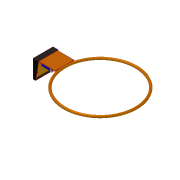
# Autodesk Inventor part: GE-12013
Saved by Autodesk Inventor 2012 (Build 160160000, 160)
## iProperties
Created: 2011-05-25
Part Number: GE-12013
Document SubType Name: Modeling
Designer: dfoster
Density: 1 g/cm^3
Description: Basketball Hoop
Mass: 471.421 g
Surface Area: 1803.58 cm^2
Volume: 471.421 cm^3
Material: Default
Title: Basketball Hoop
Author: dfoster
Autodesk Inventor part; units mm, degrees
ref_plane "YZ Plane" through (0, 0, 0) normal (1, 0, 0) x (0, 1, 0)
ref_plane "XZ Plane" through (0, 0, 0) normal (0, 1, 0) x (-1, 0, 0)
ref_plane "XY Plane" through (0, 0, 0) normal (0, 0, 1) x (1, 0, 0)
sketch "Sketch1" plane through (0, 0, 0) normal (0, 0, 1) x (1, 0, 0)
  circle A0 centre (0, 0) radius 7.9375
  line L0 (236.5375, 47.7842) -> (236.5375, -114.9552)
  dimension "d0" = 228.6
  dimension "d1" = 15.875
  constraints: 2 end point, 1 centre point, 1 coincident, 1 vertical
  measures "d0" distance edge to line of A0 L0
  measures "d1" diameter of A0
revolve "Revolution1" add sketch "Sketch1" angle 360 about axis through (236.5375, 47.7842, 0) along (0, -1, 0)
sketch "Sketch2" plane through (0, 0, 0) normal (0, 0, 1) x (1, 0, 0)
  line L0 (0, 4.7625) -> (-134.9375, 4.7625)
  line L1 (-138.1125, 1.5875) -> (-138.1125, -106.3625)
  line L2 (-138.1125, -106.3625) -> (-141.2875, -106.3625)
  line L3 (-141.2875, -106.3625) -> (-141.2875, 1.5875)
  line L4 (-134.9375, 7.9375) -> (0, 7.9375)
  line L5 (0, 7.9375) -> (0, 4.7625)
  arc A0 (-134.9375, 4.7625) -> (-138.1125, 1.5875) centre (-134.9375, 1.5875) ccw
  arc A1 (-134.9375, 7.9375) -> (-141.2875, 1.5875) centre (-134.9375, 1.5875) ccw
  point P0 (0, 0)
  point P1 (-138.1125, 4.7625)
  dimension "d5" = 0
  dimension "d6" = 7.9375
  dimension "d7" = 3.175
  dimension "d8" = 3.175
  dimension "d9" = 6.35
  dimension "d27" = 114.3
  dimension "d28" = 141.2875
  constraints: 12 end point, 4 parallel, 4 point on circle, 4 tangent, 2 centre point, 2 perpendicular, 2 point on line, 1 horizontal
  measures "d5" distance from line of point (0, 0) L5
  measures "d6" distance from line of point (0, 0) L4
  measures "d7" distance between parallel lines of L0 L4
  measures "d8" radius of A0
  measures "d9" radius of A1
  measures "d27" distance between parallel lines of L2 L4
  measures "d28" distance between parallel lines of L5 L3
extrude "Extrusion1" add sketch "Sketch2" along normal mid plane 125.4125
sketch "Sketch3" plane through (-141.2875, -106.3625, 62.7062) normal (-1, 0, 0) x (0, 0, 1)
  line L0 (0, 0) -> (0, 107.95) projected
  line L1 (0, 107.95) -> (-125.4125, 107.95) projected
  line L2 (-125.4125, 107.95) -> (-125.4125, 0) projected
  line L3 (0, 0) -> (-125.4125, 0) projected
  line L4 (0, 114.3) -> (-125.4125, 114.3) projected
  line L5 (-125.4125, 107.95) -> (-125.4125, 114.3) projected
  line L6 (0, 114.3) -> (0, 107.95) projected
  arc A0 (-103.9113, 100.9746) -> (-110.4012, 84.7629) centre (-107.1562, 92.8687) ccw
  arc A1 (-102.47, 81.5879) -> (-95.9802, 97.7996) centre (-99.2251, 89.6937) ccw
  arc A2 (-29.4323, 97.7996) -> (-22.9425, 81.5879) centre (-26.1874, 89.6937) ccw
  arc A3 (-15.0113, 84.7629) -> (-21.5012, 100.9746) centre (-18.2562, 92.8687) ccw
  arc A4 (-110.4012, 31.1246) -> (-103.9113, 14.9129) centre (-107.1562, 23.0187) ccw
  arc A5 (-95.9802, 18.0879) -> (-102.47, 34.2996) centre (-99.2251, 26.1937) ccw
  arc A6 (-22.9425, 34.2996) -> (-29.4323, 18.0879) centre (-26.1874, 26.1937) ccw
  arc A7 (-21.5012, 14.9129) -> (-15.0113, 31.1246) centre (-18.2562, 23.0187) ccw
  line L7 (-110.4012, 84.7629) -> (-102.47, 81.5879)
  line L8 (-103.9113, 100.9746) -> (-95.9802, 97.7996)
  line L9 (-21.5012, 100.9746) -> (-29.4323, 97.7996)
  line L10 (-15.0113, 84.7629) -> (-22.9425, 81.5879)
  line L11 (-22.9425, 34.2996) -> (-15.0113, 31.1246)
  line L12 (-21.5012, 14.9129) -> (-29.4323, 18.0879)
  line L13 (-103.9113, 14.9129) -> (-95.9802, 18.0879)
  line L14 (-102.47, 34.2996) -> (-110.4012, 31.1246)
  line L15 (-107.1562, 23.0187) -> (-107.1562, 92.8687)
  line L16 (-99.2251, 26.1937) -> (-99.2251, 89.6937)
  line L17 (-26.1874, 26.1937) -> (-26.1874, 89.6937)
  line L18 (-18.2562, 23.0187) -> (-18.2562, 92.8687)
  line L19 (-99.2251, 89.6937) -> (-26.1874, 89.6937)
  line L20 (-107.1562, 92.8687) -> (-18.2562, 92.8687)
  line L21 (-99.2251, 26.1937) -> (-26.1874, 26.1937)
  line L22 (-107.1562, 23.0187) -> (-18.2562, 23.0187)
  dimension "d29" = 106.3625
  dimension "d30" = 55.5752
  dimension "d31" = 87.3125
  dimension "d32" = 46.0375
  dimension "d33" = 17.4625
  dimension "d34" = 9.525
  dimension "d35" = 12.7
  dimension "d36" = 9.525
  dimension "d37" = 33.3375
  dimension "d38" = 79.375
  dimension "d39" = 34.9186
  constraints: 32 end point, 16 point on circle, 14 tangent, 8 centre point, 7 equal radius, 4 horizontal, 4 vertical, 2 parallel, 1 coincident, 1 equal length
  measures "d33" distance between parallel lines of L7 L8
  measures "d34" distance edge to line of A0 L2
  measures "d35" distance edge to line of A3 L4
  measures "d36" distance edge to line of A3 L0
  measures "d38" distance edge to line of A6 L4
hole "Hole1" at (-138.1125, -15.0812, 40.4812) direction (-1, 0, 0) diameter 6.731 end through all
pattern_linear "Rectangular Pattern1" count 2 spacing 80.9625 along (0, 0, -1) count 2 spacing 66.675 along (0, -1, 0) of "Hole1"
hole "Hole2" at (-141.2875, -49.2125, 0.7937) direction (1, 0, 0) diameter 12.7 depth 25.4 tip angle 118
sketch "Sketch4" plane through (-141.2875, -106.3625, 62.7062) normal (-1, 0, 0) x (0, 0, 1)
  line L0 (0, 0) -> (0, 107.95) projected
  line L1 (-125.4125, 107.95) -> (-125.4125, 0) projected
  line L2 (0, 0) -> (-125.4125, 0) projected
  line L3 (-128.5875, -3.175) -> (3.175, -3.175)
  line L4 (3.175, -3.175) -> (3.175, 117.475)
  line L5 (3.175, 117.475) -> (-128.5875, 117.475)
  line L6 (-128.5875, 117.475) -> (-128.5875, -3.175)
  line L7 (0, 114.3) -> (-125.4125, 114.3) projected
  line L8 (-127, 115.8875) -> (1.5875, 115.8875)
  line L9 (1.5875, 115.8875) -> (1.5875, -1.5875)
  line L10 (1.5875, -1.5875) -> (-127, -1.5875)
  line L11 (-127, -1.5875) -> (-127, 115.8875)
  point P0 (-62.7062, 106.3625)
  dimension "d49" = 3.175
  dimension "d50" = 3.175
  dimension "d51" = 3.175
  dimension "d52" = 3.175
  dimension "d53" = 1.5875
  constraints: 16 end point, 4 parallel, 2 perpendicular, 1 horizontal, 3 other
  measures "d49" distance between parallel lines of L1 L6
  measures "d50" distance between parallel lines of L0 L4
  measures "d51" distance between parallel lines of L7 L5
  measures "d52" distance between parallel lines of L2 L3
  measures "d53" distance between parallel lines of L8 L5
extrude "Extrusion2" add sketch "Sketch4" along normal blind 1.5875 contours L6 L5 L4 L3 | L8 L9 L10 L11
extrude "Extrusion3" add sketch "Sketch4" against normal blind 33.3375
sketch "Sketch8" plane through (-142.875, -109.5375, 65.8813) normal (0, 0, 1) x (1, 0, 0)
  line L0 (0, 120.65) -> (0, 0) projected
  line L1 (34.925, 0) -> (0, 0) projected
  line L2 (34.925, 0) -> (34.925, 120.65) projected
  line L3 (34.925, 120.65) -> (0, 120.65) projected
  line L4 (34.925, 114.3) -> (15.875, 0)
  line L5 (34.925, 0) -> (34.925, 114.3)
  line L6 (15.875, 0) -> (34.925, 0)
  point P0 (142.875, 109.5375)
  dimension "d67" = 6.35
  dimension "d68" = 15.875
  constraints: 6 end point, 2 perpendicular, 2 point on line
  measures "d67" distance from line of L4.start L3
  measures "d68" distance from line of L4.end L0
extrude "Extrusion7" cut sketch "Sketch8" against normal through all contours L4 L2 L1
sketch "Sketch5" plane through (-141.2875, -49.2125, 0.7937) normal (1, 0, 0) x (0, 0, -1)
  circle A0 centre (0, 0) radius 6.35 projected
  circle A1 centre (0, 0) radius 4.7625
  point P0 (0.7937, 49.2125)
  dimension "d58" = 9.525
  constraints: 1 centre point, 1 coincident
  measures "d58" diameter of A1
extrude "Extrusion4" add sketch "Sketch5" along normal blind 60.325 contours A1
sketch "Sketch6" plane through (-80.9625, -49.2125, 0.7937) normal (1, 0, 0) x (0, 0, -1)
  circle A0 centre (0, 0) radius 4.7625 projected
  circle A1 centre (0, 0) radius 19.05
  point P0 (0.7937, 49.2125)
  dimension "d61" = 38.1
  constraints: 1 centre point, 1 coincident
  measures "d61" diameter of A1
extrude "Extrusion5" add sketch "Sketch6" along normal blind 1.905
sketch "Sketch7" plane through (-79.0575, -49.2125, 0.7937) normal (1, 0, 0) x (0, 0, -1)
  circle A0 centre (0, 0) radius 4.7625 projected
  circle A1 centre (0, 0) radius 19.05 projected
  line L0 (0, 10.9985) -> (9.525, 5.4993)
  line L1 (9.525, 5.4993) -> (9.525, -5.4993)
  line L2 (9.525, -5.4993) -> (0, -10.9985)
  line L3 (0, -10.9985) -> (-9.525, -5.4993)
  line L4 (-9.525, -5.4993) -> (-9.525, 5.4993)
  line L5 (-9.525, 5.4993) -> (0, 10.9985)
  point P0 (0.7937, 49.2125)
  dimension "d64" = 19.05
  constraints: 12 end point, 1 coincident, 13 other
  measures "d64" distance between parallel lines of L3 L0
extrude "Extrusion6" add sketch "Sketch7" along normal blind 6.35 contours L0 L1 L2 L3 L4 L5
sketch "Sketch9" plane through (-138.1125, -106.3625, 62.7062) normal (1, 0, 0) x (0, 0, -1)
  circle A0 centre (61.9125, 57.15) radius 6.35 projected
  circle A1 centre (61.9125, 57.15) radius 15.0812
  circle A2 centre (61.9125, 57.15) radius 8.7313
  point P0 (62.7062, 106.3625)
  dimension "d71" = 30.1625
  dimension "d72" = 17.4625
  constraints: 2 centre point, 1 coincident, 1 concentric
  measures "d71" diameter of A1
  measures "d72" diameter of A2
extrude "Extrusion8" add sketch "Sketch9" along normal blind 57.15 contours A1
equation "\"d50\" = d49"
equation "\"d51\" = d49"
equation "\"d52\" = d49"
body "Solid1"
